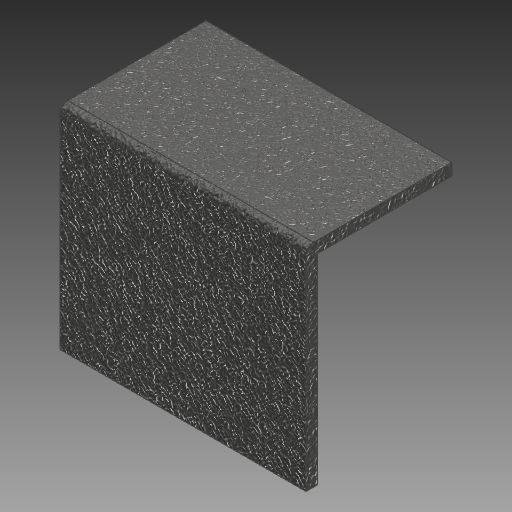
# Autodesk Inventor part: ZAŚLEPKA PRZEDNIA DOLNA CZARNEJ OBUDOWY STOJAKA
Saved by Autodesk Inventor 2017 SP1 (Build 210196100, 196)
## iProperties
Created: 2020-12-27
Part Number: ZAŚLEPKA PRZEDNIA DOLNA CZARNEJ OBUDOWY STOJAKA
Material: Tworzywo sztuczne, nieprzezroczyste czarne
Document SubType Name: Modeling
Designer: Napoleon
Mass: 2.05291 g
Surface Area: 31.0142 cm^2
Volume: 2.15641 cm^3
Density: 0.952 g/cm^3
Appearance: Chropowaty, teksturowany - czarny
Author: Napoleon
Autodesk Inventor part; units mm, degrees
ref_plane "YZ Plane" through (0, 0, 0) normal (1, 0, 0) x (0, 1, 0)
ref_plane "XZ Plane" through (0, 0, 0) normal (0, 1, 0) x (-1, 0, 0)
sketch "Szkic1" plane through (0, 0, 0) normal (0, 0, 1) x (1, 0, 0)
  line L0 (16, -77.5) -> (-16, -77.5)
  line L1 (-16, -77.5) -> (-16, -96.5)
  line L2 (-16, -96.5) -> (16, -96.5)
  line L3 (16, -96.5) -> (16, -77.5)
  point P0 (0, 0)
  dimension "d1" = 32
  constraints: 8 end point, 2 perpendicular, 1 horizontal, 1 vertical
  measures "d1" distance of L0.start L0.end
extrude "Wyciągnięcie proste1" add sketch "Szkic1" against normal blind 1.5
sketch "Szkic2" plane through (0, 0, -1.5) normal (0, 0, -1) x (-1, 0, 0)
  line L0 (-16, -77.5) -> (-16, -96.5) projected
  line L1 (16, -96.5) -> (-16, -96.5)
  line L2 (-16, -96.5) -> (-16, -95)
  line L3 (-16, -95) -> (16, -95)
  line L4 (16, -95) -> (16, -96.5)
  point P0 (0, 0)
  dimension "d5" = 1.5
  constraints: 8 end point, 2 parallel, 1 horizontal, 1 perpendicular, 1 point on line
  measures "d5" distance of L1.end L2.end
ref_plane "Płaszczyzna konstrukcyjna1" through (-22.5, -96.5, -27.5684) normal (0, 0, -1) x (0, 1, 0)
extrude "Wyciągnięcie proste2" add sketch "Szkic2" along normal up to surface (26.0684 mm away)
fillet "Zaokrąglenie1" radius 1 1 edges at (0, -96.5, 0)
